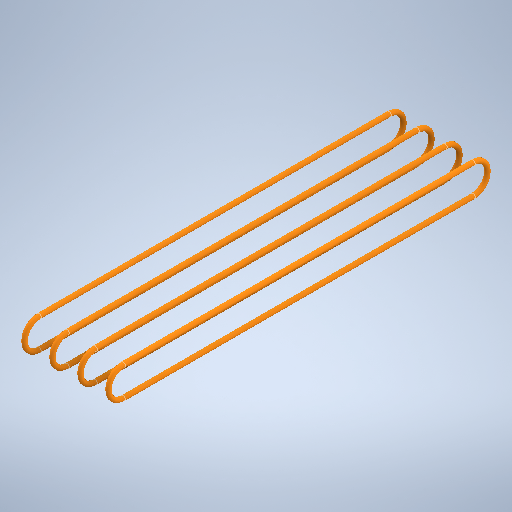
# Autodesk Inventor part: ball_loading_v1_circle_B
Saved by Autodesk Inventor 2025.1 (Build 291241000, 241)
## iProperties
Created: 2024-11-12
Part Number: ball_loading_v1_circle_B
Material: ゴム
Document SubType Name: Modeling
Designer: haruy
Density: 0.93 g/cm^3
Appearance: オレンジ
Author: haruy
Autodesk Inventor part; units mm, degrees
ref_plane "XZ Plane" through (0, 0, 0) normal (0, 1, 0) x (-1, 0, 0)
ref_plane "XY Plane" through (0, 0, 0) normal (0, 0, 1) x (1, 0, 0)
sketch "スケッチ1" plane through (0, 0, 0) normal (1, 0, 0) x (0, 1, 0)
  line L0 (12.5, 0) -> (12.5, -300)
  line L1 (-12.5, 0) -> (-12.5, -300)
  arc A0 (12.5, 0) -> (-12.5, 0) centre (0, 0) ccw
  arc A1 (-12.5, -300) -> (12.5, -300) centre (0, -300) ccw
  circle A2 centre (0, 0) radius 10.5
  circle A3 centre (0, -300) radius 10.5
  point P0 (10.5, -300)
  point P1 (-10.5, -300)
  point P2 (-10.5, 0)
  point P3 (10.5, 0)
  dimension "d7" = 12.5
  dimension "d8" = 12.5
  dimension "d14" = 21
  dimension "d15" = 21
  dimension "d18" = 300
  dimension "d19" = 0
  constraints: 4 centre point, 4 end point, 4 point on circle, 2 coincident
  measures "d7" radius of A0
  measures "d8" radius of A1
  measures "d14" diameter of A2
  measures "d15" diameter of A3
  measures "d18" distance of A1.centre A0.centre
  measures "d19" distance of point (0, 0) A0.centre
sketch "スケッチ2" plane through (0, 0, 0) normal (0, 0, 1) x (1, 0, 0)
  circle A0 centre (0, 12.5) radius 2
  point P0 (0, 0)
  dimension "d4" = 4
  dimension "d5" = 12.5
  dimension "d6" = 0
  constraints: 1 centre point
  measures "d4" diameter of A0
  measures "d5" distance of A0.centre point (0, 0)
  measures "d6" horizontal distance of point (0, 0) A0.centre
sweep "スイープ1" add profiles "スケッチ2" path "スケッチ1" path curves L0 A1 L1 A0
pattern_linear "矩形状パターン1" count 4 spacing 24 along (1, 0, 0)
extrude "押し出し1" add sketch "スケッチ1" along normal blind 10 separate body contours L0 A1 L1 A0 | A2 | A3
equation "\"d8\" = d7"
